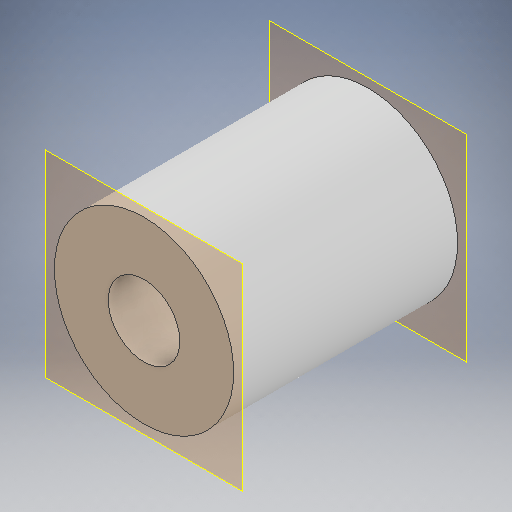
# Autodesk Inventor part: shaft_coupler 5mm_to_8mm
Saved by Autodesk Inventor 2025.2 (Build 292293000, 293)
## iProperties
Created: 2025-04-06
Part Number: shaft_coupler 5mm_to_8mm
Material: Generic
Document SubType Name: Modeling
Designer: Tiago
Density: 1 g/cm^3
Appearance: Default
Author: Tiago
Autodesk Inventor part; units mm, degrees
ref_plane "YZ Plane" through (0, 0, 0) normal (1, 0, 0) x (0, 1, 0)
ref_plane "XZ Plane" through (0, 0, 0) normal (0, 1, 0) x (-1, 0, 0)
sketch "Sketch1" plane through (0, 0, 0) normal (0, 0, 1) x (1, 0, 0)
  circle A0 centre (0, 0) radius 10
  circle A1 centre (0, 0) radius 2.5
  dimension "D" = 20
  dimension "di1" = 5
  constraints: 2 centre point, 2 coincident
  measures "D" diameter of A0
  measures "di1" diameter of A1
ref_plane "Work Plane1" through (0, 0, 25) normal (0, 0, 1) x (1, 0, 0)
sketch "Sketch2" plane through (0, 0, 25) normal (0, 0, 1) x (1, 0, 0)
  circle A0 centre (0, 0) radius 4
  circle A1 centre (0, 0) radius 10
  dimension "di2" = 8
  dimension "d4" = 20
  constraints: 2 centre point, 2 coincident
  measures "di2" diameter of A0
  measures "d4" diameter of A1
extrude "Extrusion1" add sketch "Sketch2" against normal up to surface (25 mm away)
extrude "Extrusion2" add sketch "Sketch1" along normal blind 10
equation "\"d4\" = D"
body "Solid2"
